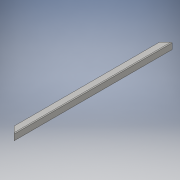
# Autodesk Inventor part: Chasis 28 piece
Saved by Autodesk Inventor 2016 (Build 200138000, 138)
## iProperties
Created: 2016-01-16
Part Number: Chasis 28 piece
Material: Generic
Document SubType Name: Modeling
Designer: 17thorpc
Density: 1 g/cm^3
Appearance: Default
Author: 17thorpc
Autodesk Inventor part; units mm, degrees
ref_plane "YZ Plane" through (0, 0, 0) normal (1, 0, 0) x (0, 1, 0)
ref_plane "XZ Plane" through (0, 0, 0) normal (0, 1, 0) x (-1, 0, 0)
ref_plane "XY Plane" through (0, 0, 0) normal (0, 0, 1) x (1, 0, 0)
sketch "Sketch1" plane through (0, 0, 0) normal (0, 0, 1) x (1, 0, 0)
  line L0 (0, 0) -> (25.4, 0)
  line L1 (28.575, 3.175) -> (28.575, 28.575)
  line L2 (25.4, 31.75) -> (0, 31.75)
  line L3 (0, 31.75) -> (0, 28.575)
  line L4 (0, 28.575) -> (25.4, 28.575)
  line L5 (25.4, 28.575) -> (25.4, 3.175)
  line L6 (25.4, 3.175) -> (0, 3.175)
  line L7 (0, 3.175) -> (0, 0)
  arc A0 (28.575, 28.575) -> (25.4, 31.75) centre (25.4, 28.575) ccw
  arc A1 (25.4, 0) -> (28.575, 3.175) centre (25.4, 3.175) ccw
  point P0 (28.575, 0)
  point P1 (28.575, 31.75)
  dimension "d0" = 28.575
  dimension "d1" = 31.75
  dimension "d2" = 3.175
  dimension "d3" = 25.4
  dimension "d4" = 25.4
  dimension "d5" = 3.175
  constraints: 16 end point, 6 perpendicular, 5 point on line, 4 point on circle, 4 tangent, 2 centre point, 1 equal radius, 1 horizontal, 1 parallel
  measures "d0" distance of L0.start point (28.575, 0)
  measures "d1" distance of point (28.575, 0) point (28.575, 31.75)
  measures "d2" distance of L2.end L3.end
  measures "d3" distance of L3.end L4.end
  measures "d4" distance of L4.end L5.end
  measures "d5" radius of A0
extrude "Extrusion1" add sketch "Sketch1" along normal blind 711.2
sketch "Sketch2" plane through (0, 31.75, 0) normal (0, 1, 0) x (1, 0, 0)
  line L0 (25.4, 0) -> (28.575, 0) projected
  line L1 (25.4, 0) -> (28.575, 0)
  line L2 (28.575, 0) -> (0, -28.575)
  line L3 (0, 0) -> (0, -711.2) projected
  line L4 (0, -28.575) -> (0, 0)
  line L5 (0, 0) -> (28.575, 0)
  dimension "d8" = 45
  constraints: 8 end point, 2 horizontal, 1 vertical
  measures "d8" angle of L1 L2
extrude "Extrusion2" cut sketch "Sketch2" against normal blind 711.2
sketch "Sketch3" plane through (0, 31.75, 711.2) normal (0, 1, 0) x (1, 0, 0)
  line L0 (0, 0) -> (25.4, 0) projected
  line L1 (25.4, 0) -> (28.575, 0) projected
  line L2 (25.4, 0) -> (28.575, 0)
  line L3 (28.575, 0) -> (0, 28.575)
  line L4 (0, 682.625) -> (0, 0) projected
  line L5 (0, 28.575) -> (0, 0)
  line L6 (0, 0) -> (28.575, 0)
  point P0 (0, 711.2)
  dimension "d11" = 45
  constraints: 8 end point, 2 collinear, 1 horizontal
  measures "d11" angle of L3 L2
extrude "Extrusion3" cut sketch "Sketch3" against normal blind 711.2
body "Solid1"
